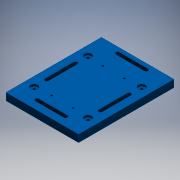
# Autodesk Inventor part: sCMOSmountingBase
Saved by Autodesk Inventor 2016 (Build 200138000, 138)
## iProperties
Created: 2016-02-19
Part Number: sCMOSmountingBase
Material: Generic
Document SubType Name: Modeling
Designer: sims01
Density: 1 g/cm^3
Appearance: Default
Author: sims01
Autodesk Inventor part; units mm, degrees
ref_plane "YZ Plane" through (0, 0, 0) normal (1, 0, 0) x (0, 1, 0)
ref_plane "XZ Plane" through (0, 0, 0) normal (0, 1, 0) x (-1, 0, 0)
ref_plane "XY Plane" through (0, 0, 0) normal (0, 0, 1) x (1, 0, 0)
sketch "Sketch2" plane through (0, 0, 0) normal (0, 0, 1) x (1, 0, 0)
  line L0 (-42.5, 62.5) -> (42.5, 62.5)
  line L1 (42.5, 62.5) -> (42.5, -62.5)
  line L2 (42.5, -62.5) -> (-42.5, -62.5)
  line L3 (-42.5, -62.5) -> (-42.5, 62.5)
  line L4 (-67.5, 92.5) -> (67.5, 92.5)
  line L5 (67.5, 92.5) -> (67.5, -85)
  line L6 (67.5, -85) -> (-67.5, -85)
  line L7 (-67.5, -85) -> (-67.5, 92.5)
  point P0 (0, 0)
  dimension "d16" = 125
  dimension "d17" = 62.5
  dimension "d18" = 85
  dimension "d19" = 42.5
  dimension "d20" = 25
  dimension "d21" = 25
  dimension "d23" = 22.5
  dimension "d75" = 30
  constraints: 16 end point, 4 parallel, 2 horizontal, 2 perpendicular
  measures "d16" distance of L0.end L1.end
  measures "d17" distance from line of point (0, 0) L0
  measures "d18" distance of L0.start L0.end
  measures "d19" distance from line of point (0, 0) L3
  measures "d20" distance between parallel lines of L5 L1
  measures "d21" distance between parallel lines of L7 L3
  measures "d23" distance between parallel lines of L6 L2
  measures "d75" distance between parallel lines of L4 L0
extrude "flash4base" add sketch "Sketch2" along normal blind 13.5 contours L0 L1 L2 L3 | L4 L5 L6 L7
sketch "Sketch3" plane through (0, 0, 0) normal (0, 0, -1) x (-1, 0, 0)
  point P0 (0, 0)
  point P1 (-20, 47.65)
  point P2 (20, 47.65)
  point P3 (-20, -47.65)
  point P4 (20, -47.65)
  dimension "d26" = 40
  dimension "d27" = 20
  dimension "d28" = 95.3
  dimension "d29" = 47.65
  constraints: 2 horizontal alignment, 2 vertical alignment
  measures "d26" distance of point (20, 47.65) point (-20, 47.65)
  measures "d27" horizontal distance of point (0, 0) point (20, 47.65)
  measures "d28" distance of point (20, -47.65) point (20, 47.65)
  measures "d29" vertical distance of point (0, 0) point (20, 47.65)
hole "flash4mountingholes" at (20, 47.65, 0) at (-20, 47.65, 0) at (20, -47.65, 0) at (-20, -47.65, 0) direction (0, 0, 1) diameter 3.4 end through all counterbore diameter 11 counterbore depth 2.6 clearance for "Hex Head Cap Screw ISO 24017" size "M3" standard "ISO"
sketch "Sketch4" plane through (0, 0, 13.5) normal (0, 0, 1) x (1, 0, 0)
  point P0 (0, 0)
  point P1 (50, -50)
  point P2 (-50, -50)
  point P3 (50, 50)
  point P4 (-50, 50)
  dimension "d37" = 100
  dimension "d38" = 50
  dimension "d39" = 100
  dimension "d56" = 50
  constraints: 2 horizontal alignment, 2 vertical alignment
  measures "d37" distance of point (-50, -50) point (50, -50)
  measures "d38" horizontal distance of point (-50, -50) point (0, 0)
  measures "d39" distance of point (-50, 50) point (-50, -50)
  measures "d56" horizontal distance of point (0, 0) point (-50, 50)
hole "mountinPostMountingHoles" at (50, -50, 13.5) at (-50, -50, 13.5) at (50, 50, 13.5) at (-50, 50, 13.5) direction (0, 0, -1) diameter 4.5 end through all counterbore diameter 13 counterbore depth 3.4 clearance for "Hex Head Cap Screw ISO 24017" size "M4" standard "ISO"
sketch "Sketch5" plane through (0, 0, 13.5) normal (0, 0, 1) x (1, 0, 0)
  line L0 (-50.3, 30) -> (-48.7, 30)
  line L1 (-46.7, 28) -> (-46.7, -27)
  line L2 (-49.7, -30) -> (-50.3, -30)
  line L3 (-53.3, -27) -> (-53.3, 27)
  line L4 (49.7, 30) -> (50.3, 30)
  line L5 (53.3, 27) -> (53.3, -27)
  line L6 (50.3, -30) -> (49.7, -30)
  line L7 (46.7, -27) -> (46.7, 27)
  arc A0 (-46.7, 28) -> (-48.7, 30) centre (-48.7, 28) ccw
  arc A1 (-50.3, 30) -> (-53.3, 27) centre (-50.3, 27) ccw
  arc A2 (-53.3, -27) -> (-50.3, -30) centre (-50.3, -27) ccw
  arc A3 (-49.7, -30) -> (-46.7, -27) centre (-49.7, -27) ccw
  arc A4 (46.7, -27) -> (49.7, -30) centre (49.7, -27) ccw
  arc A5 (50.3, -30) -> (53.3, -27) centre (50.3, -27) ccw
  arc A6 (49.7, 30) -> (46.7, 27) centre (49.7, 27) ccw
  arc A7 (53.3, 27) -> (50.3, 30) centre (50.3, 27) ccw
  line L8 (-27, 85) -> (27, 85)
  line L9 (30, 82) -> (30, 81.4)
  line L10 (27, 78.4) -> (-27, 78.4)
  line L11 (-30, 81.4) -> (-30, 82)
  line L12 (-27, -65) -> (27, -65)
  line L13 (30, -68) -> (30, -68.6)
  line L14 (27, -71.6) -> (-27, -71.6)
  line L15 (-30, -68.6) -> (-30, -68)
  arc A8 (-27, 85) -> (-30, 82) centre (-27, 82) ccw
  arc A9 (-30, 81.4) -> (-27, 78.4) centre (-27, 81.4) ccw
  arc A10 (30, 82) -> (27, 85) centre (27, 82) ccw
  arc A11 (27, 78.4) -> (30, 81.4) centre (27, 81.4) ccw
  arc A12 (-27, -65) -> (-30, -68) centre (-27, -68) ccw
  arc A13 (-30, -68.6) -> (-27, -71.6) centre (-27, -68.6) ccw
  arc A14 (30, -68) -> (27, -65) centre (27, -68) ccw
  arc A15 (27, -71.6) -> (30, -68.6) centre (27, -68.6) ccw
  point P0 (0, 0)
  point P1 (46.7, 30)
  point P2 (53.3, 30)
  point P3 (-30, -71.6)
  dimension "d48" = 6.6
  dimension "d50" = 6.6
  dimension "d52" = 30
  dimension "d53" = 30
  dimension "d54" = 30
  dimension "d55" = 30
  dimension "d57" = 2
  dimension "d58" = 3
  dimension "d59" = 3
  dimension "d62" = 6.6
  dimension "d63" = 6.6
  dimension "d64" = 30
  dimension "d65" = 30
  dimension "d66" = 30
  dimension "d67" = 30
  dimension "d70" = 3
  dimension "d71" = 93.4
  dimension "d72" = 46.7
  dimension "d73" = 143.4
  dimension "d74" = 65
  constraints: 32 end point, 32 point on circle, 32 tangent, 16 centre point, 12 equal radius, 8 parallel, 6 point on line, 4 horizontal, 4 perpendicular
  measures "d48" distance between parallel lines of L3 L1
  measures "d50" distance of point (46.7, 30) point (53.3, 30)
  measures "d52" distance from line of point (0, 0) L4
  measures "d53" distance from line of point (0, 0) L6
  measures "d54" distance from line of point (0, 0) L0
  measures "d55" distance from line of L2 point (0, 0)
  measures "d57" radius of A0
  measures "d58" radius of A1
  measures "d59" radius of A2
  measures "d62" distance between parallel lines of L14 L12
  measures "d63" distance between parallel lines of L10 L8
  measures "d64" distance from line of point (0, 0) L9
  measures "d65" distance from line of L11 point (0, 0)
  measures "d66" horizontal distance of point (-30, -71.6) point (0, 0)
  measures "d67" distance from line of point (0, 0) L13
  measures "d70" radius of A8
  measures "d71" distance between parallel lines of L7 L1
  measures "d72" distance from line of point (0, 0) L7
  measures "d73" distance between parallel lines of L12 L10
  measures "d74" distance from line of L12 point (0, 0)
extrude "m6Alignment" cut sketch "Sketch5" against normal through all
equation "\"d17\" = 0.5 * d16"
equation "\"d19\" = 0.5 * d18"
equation "\"d27\" = 0.5 * d26"
equation "\"d29\" = 0.5 * d28"
equation "\"d38\" = 0.5 * d37"
equation "\"d56\" = 0.5 * d39"
equation "\"d53\" = d52"
equation "\"d54\" = d52"
equation "\"d55\" = d54"
equation "\"d62\" = d50"
equation "\"d63\" = d50"
equation "\"d64\" = d52"
equation "\"d65\" = d64"
equation "\"d66\" = d65"
equation "\"d67\" = d64"
equation "\"d72\" = 0.5 * d71"
equation "\"d10\" = 125"
equation "\"d11\" = 7"
equation "\"d12\" = 4"
body "Solid1"
